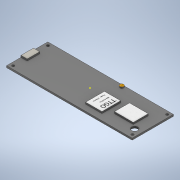
# Autodesk Inventor part: tBeam
Saved by Autodesk Inventor 2020 (Build 240168000, 168)
## iProperties
Created: 2022-02-21
Part Number: tBeam
Material: Genérico
Document SubType Name: Modeling
Designer: DANIEL
Density: 1 g/cm^3
Appearance: Suave - Negro
Author: DANIEL
Autodesk Inventor part; units mm, degrees
ref_plane "YZ Plane" through (0, 0, 0) normal (1, 0, 0) x (0, 1, 0)
ref_plane "XZ Plane" through (0, 0, 0) normal (0, 1, 0) x (-1, 0, 0)
ref_plane "XY Plane" through (0, 0, 0) normal (0, 0, 1) x (1, 0, 0)
sketch "Boceto1" plane through (0, 0, 0) normal (0, 1, 0) x (-1, 0, 0)
  line L0 (50.065, 16.445) -> (-50.065, 16.445)
  line L1 (-50.065, 16.445) -> (-50.065, -16.445)
  line L2 (-50.065, -16.445) -> (50.065, -16.445)
  line L3 (50.065, -16.445) -> (50.065, 16.445)
  point P0 (0, 0)
  dimension "q" = 100.13
  dimension "t" = 32.89
  dimension "d3" = 16.445
  dimension "d4" = 50.065
  constraints: 8 end point, 2 parallel, 1 horizontal, 1 perpendicular
  measures "q" distance of L2.end L1.end
  measures "t" distance of L1.end L0.end
  measures "d3" distance from line of point (0, 0) L0
  measures "d4" distance from line of point (0, 0) L3
extrude "Extrusión1" add sketch "Boceto1" along normal blind 1.4
sketch "Boceto2" plane through (0, 1.4, 0) normal (0, 1, 0) x (1, 0, 0)
  circle A0 centre (-47.395, -13.855) radius 1
  circle A1 centre (-47.395, 13.855) radius 1
  line L0 (-50.065, -16.445) -> (50.065, -16.445) projected
  line L1 (50.065, 16.445) -> (-50.065, 16.445) projected
  line L2 (-50.065, 16.445) -> (-50.065, -16.445) projected
  circle A2 centre (47.705, -13.855) radius 1
  circle A3 centre (47.705, 13.855) radius 1
  line L3 (50.065, -16.445) -> (50.065, 16.445) projected
  point P0 (0, 0)
  dimension "d7" = 2
  dimension "d8" = 2
  dimension "v" = 2.59
  dimension "d10" = 2.59
  dimension "d11" = 2.67
  dimension "d12" = 2.67
  dimension "d13" = 2
  dimension "d14" = 2
  dimension "d15" = 2.59
  dimension "d16" = 2.59
  dimension "d17" = 2.36
  dimension "d18" = 2.36
  constraints: 4 centre point
  measures "d7" diameter of A0
  measures "d8" diameter of A1
  measures "v" distance from line of L0 A0.centre
  measures "d10" distance from line of L1 A1.centre
  measures "d11" distance from line of L2 A0.centre
  measures "d12" distance from line of L2 A1.centre
  measures "d13" diameter of A2
  measures "d14" diameter of A3
  measures "d15" distance from line of L0 A2.centre
  measures "d16" distance from line of L1 A3.centre
  measures "d17" distance from line of A2.centre L3
  measures "d18" distance from line of A3.centre L3
extrude "Extrusión2" cut sketch "Boceto2" against normal blind 1.4 contours A0 | A1 | A2 | A3
sketch "Boceto3" plane through (0, 1.4, 0) normal (0, 1, 0) x (1, 0, 0)
  line L0 (-50.065, 16.445) -> (-50.065, -16.445) projected
  line L1 (-45.065, -5.0075) -> (-50.065, -5.0075)
  line L2 (-50.065, -5.0075) -> (-50.065, 4.9925)
  line L3 (-50.065, 4.9925) -> (-45.065, 4.9925)
  line L4 (-45.065, 4.9925) -> (-45.065, -5.0075)
  line L5 (8.065, -11.555) -> (21.065, -11.555)
  line L6 (21.065, -11.555) -> (21.065, 3.445)
  line L7 (21.065, 3.445) -> (8.065, 3.445)
  line L8 (8.065, 3.445) -> (8.065, -11.555)
  line L9 (50.065, -16.445) -> (50.065, 16.445) projected
  line L10 (50.065, 16.445) -> (-50.065, 16.445) projected
  line L11 (41.065, -6.555) -> (26.065, -6.555)
  line L12 (26.065, -6.555) -> (26.065, 5.445)
  line L13 (26.065, 5.445) -> (41.065, 5.445)
  line L14 (41.065, 5.445) -> (41.065, -6.555)
  point P0 (0, 0)
  dimension "d22" = 10
  dimension "d23" = 5
  dimension "d24" = 13
  dimension "d25" = 15
  dimension "d26" = 42
  dimension "d27" = 28
  dimension "d28" = 15
  dimension "d29" = 12
  dimension "d30" = 24
  dimension "d31" = 23
  constraints: 24 end point, 6 parallel, 3 horizontal, 3 perpendicular, 1 point on line
  measures "d22" distance between parallel lines of L3 L1
  measures "d23" distance between parallel lines of L0 L4
  measures "d24" distance of L7.end L6.end
  measures "d25" distance of L6.end L5.end
  measures "d26" distance between parallel lines of L9 L8
  measures "d27" distance between parallel lines of L10 L5
  measures "d28" distance of L12.end L13.end
  measures "d29" distance of L11.end L12.end
  measures "d30" distance between parallel lines of L12 L9
  measures "d31" distance between parallel lines of L10 L11
extrude "Extrusión3" add sketch "Boceto3" along normal blind 1.4
sketch "Boceto4" plane through (0, 2.8, 0) normal (0, 1, 0) x (1, 0, 0)
  point P0 (0, 0)
  point P1 (8.9547, -10.1632)
sketch "Boceto5" plane through (0, 2.8, 0) normal (0, 1, 0) x (1, 0, 0)
  line L0 (19.4822, 1.7557) -> (19.4822, -9.7421) construction
  line L1 (19.4822, -9.7421) -> (15.3355, -9.7421) construction
  line L2 (15.3355, -9.7421) -> (15.3355, 1.7557) construction
  line L3 (15.3355, 1.7557) -> (19.4822, 1.7557) construction
  point P0 (0, 0)
  constraints: 2 other
sketch "Boceto6" plane through (0, 2.8, 0) normal (0, 1, 0) x (1, 0, 0)
  line L0 (14.4245, 1.2531) -> (14.4245, -8.6603) construction
  line L1 (14.4245, -8.6603) -> (9.5235, -8.6603) construction
  line L2 (9.5235, -8.6603) -> (9.5235, 1.2531) construction
  line L3 (9.5235, 1.2531) -> (14.4245, 1.2531) construction
  point P0 (0, 0)
  constraints: 2 other
sketch "Boceto7" plane through (0, 1.4, 0) normal (0, 1, 0) x (1, 0, 0)
  circle A0 centre (44.565, -8.945) radius 2.5
  line L0 (50.065, -16.445) -> (50.065, 16.445) projected
  line L1 (-50.065, -16.445) -> (50.065, -16.445) projected
  point P0 (0, 0)
  dimension "d34" = 5
  dimension "d38" = 3
  dimension "d39" = 5
  constraints: 1 centre point
  measures "d34" diameter of A0
  measures "d38" distance edge to line of A0 L0
  measures "d39" distance edge to line of A0 L1
extrude "Extrusión4" cut sketch "Boceto7" against normal blind 1.4
sketch "Boceto8" plane through (0, 1.4, 0) normal (0, 1, 0) x (1, 0, 0)
  circle A0 centre (10.565, 14.8534) radius 1.5
  line L0 (50.065, -16.445) -> (50.065, 16.445) projected
  point P0 (0, 0)
  dimension "d42" = 3
  dimension "d43" = 41
  constraints: 1 centre point
  measures "d42" diameter of A0
extrude "Extrusión5" add sketch "Boceto8" along normal blind 1
equation "\"d3\" = 0.5 * t"
equation "\"d4\" = 0.5 * q"
equation "\"d10\" = v"
equation "\"d15\" = v"
equation "\"d16\" = v"
